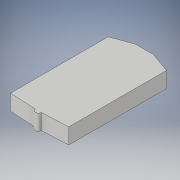
# Autodesk Inventor part: chassis_plate_v7
Saved by Autodesk Inventor 2019 (Build 230136000, 136)
## iProperties
Created: 2020-02-10
Part Number: chassis_plate_v7
Material: Generic
Document SubType Name: Modeling
Designer: close
Density: 1 g/cm^3
Appearance: Default
Author: close
Autodesk Inventor part; units mm, degrees
ref_plane "YZ Plane" through (0, 0, 0) normal (1, 0, 0) x (0, 1, 0)
ref_plane "XZ Plane" through (0, 0, 0) normal (0, 1, 0) x (-1, 0, 0)
ref_plane "XY Plane" through (0, 0, 0) normal (0, 0, 1) x (1, 0, 0)
sketch "Sketch2" plane through (0, 0, 0) normal (0, 1, 0) x (-1, 0, 0)
  line L0 (65, -3.0659) -> (65, -220.6213)
  line L1 (65, -220.6213) -> (20, -237)
  line L2 (20, -237) -> (-20, -237)
  line L3 (-20, -237) -> (-65, -220.6213)
  line L4 (-65, -220.6213) -> (-65, -3.0659)
  line L5 (65, -3.0659) -> (6.5, 0)
  line L6 (-65, -3.0659) -> (-6.5, 0)
  arc A0 (6.5, 0) -> (-6.5, 0) centre (0, 0) ccw
  line L7 (16, -233) -> (-16, -233) construction
  line L8 (6.5, 0) -> (-6.5, 0) construction
  dimension "d0" = 130
  dimension "d1" = 32
  dimension "d4" = 65
  dimension "d5" = 0
  dimension "d6" = 6.5
  dimension "d7" = 93
  dimension "d9" = 4
  dimension "d11" = 237
  dimension "d12" = 160
  dimension "d28" = 40
  dimension "d30" = 4
  dimension "d31" = 160
  dimension "d93" = 93
  dimension "d95" = 20
  constraints: 18 end point, 4 coincident, 2 perpendicular, 2 point on circle, 1 centre point, 1 horizontal, 1 parallel, 1 vertical
  measures "d0" distance between parallel lines of L4 L0
  measures "d1" distance of point (-16, -233) point (16, -233)
  measures "d4" distance from line of point (0, 0) L0
  measures "d5" distance from line of point (0, 0) L8
  measures "d6" radius of A0
  measures "d7" angle of L0 L5
  measures "d9" distance between parallel lines of L2 L7
  measures "d11" distance from line of L2 point (0, 0)
  measures "d12" angle of L2 L1
  measures "d28" distance of L1.end L2.end
  measures "d30" horizontal distance of L1.end point (16, -233)
  measures "d31" angle of L3 L2
  measures "d93" angle of L4 L6
  measures "d95" horizontal distance of point (0, 0) L1.end
extrude "Extrusion3" add sketch "Sketch2" along normal blind 35
shell "Shell1" thickness 2.5 removed faces 1 at (45.5, 0, -74.5624)
equation "\"d4\" = 0.5 * d0"
body "Solid2"
